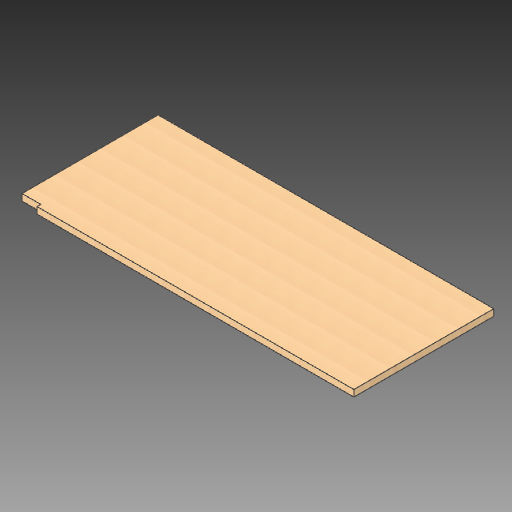
# Autodesk Inventor part: Причал фанера
Saved by Autodesk Inventor 2019 (Build 230136000, 136)
## iProperties
Created: 2018-10-10
Part Number: Причал фанера
Material: Ясень
Document SubType Name: Modeling
Designer: Андреев Н.Л.
Density: 0.641 g/cm^3
Appearance: Дверь — ясень
ШИРИНА: 371
ДЛИНА: 890
ТОЛЩВЫС: 17
Author: Андреев Н.Л.
Autodesk Inventor part; units mm, degrees
ref_plane "YZ Plane" through (0, 0, 0) normal (1, 0, 0) x (0, 1, 0)
ref_plane "XZ Plane" through (0, 0, 0) normal (0, 1, 0) x (-1, 0, 0)
ref_plane "XY Plane" through (0, 0, 0) normal (0, 0, 1) x (1, 0, 0)
sketch "Эскиз1" plane through (0, 0, 0) normal (0, 1, 0) x (-1, 0, 0)
  line L0 (0, 0) -> (890, 0)
  line L1 (890, 0) -> (890, 371)
  line L2 (890, 371) -> (0, 371)
  line L3 (0, 371) -> (0, 0)
  dimension "ШИРИНА" = 371
  dimension "ДЛИНА" = 890
  constraints: 8 end point, 2 parallel, 1 horizontal, 1 perpendicular
  measures "ШИРИНА" distance between parallel lines of L2 L0
  measures "ДЛИНА" distance between parallel lines of L3 L1
extrude "Выдавливание1" add sketch "Эскиз1" against normal blind 17.4
sketch "Эскиз2" plane through (-890, 0, 371) normal (0, 0, 1) x (1, 0, 0)
  line L0 (0, 0) -> (890, 0) construction
  line L1 (0, 0) -> (0, -17.4) construction
  line L2 (890, -17.4) -> (0, -17.4) construction
  line L3 (890, 0) -> (890, -17.4) construction
  line L4 (0, 0) -> (50, 0)
  line L5 (50, 0) -> (50, -17.4)
  line L6 (50, -17.4) -> (0, -17.4)
  line L7 (0, -17.4) -> (0, 0)
  point P0 (890, 0)
  dimension "d4" = 50
  constraints: 8 end point, 2 parallel, 1 horizontal, 1 perpendicular, 1 point on line
  measures "d4" distance of L5.end L6.end
extrude "Выдавливание2" cut sketch "Эскиз2" against normal blind 10
equation "\"ДЛИНА\" = пДлПроступи - пОтступПодступ"
equation "\"ТОЛЩВЫС\" = пТолПодступенка"
equation "\"d4\" = пОтступШипа"
equation "\"d5\" = пШипПодступ"
equation "\"пДлПроступи\" = 900"
equation "\"пПодъем\" = 162.5"
equation "\"пХод\" = 296.8"
equation "\"пЭффШаг\" = 621.8"
equation "\"пСвес\" = 30.2"
equation "\"пОтступСтен\" = 5"
equation "\"пДиаг\" = 338.3733"
equation "\"пШирПроступи\" = 327"
equation "\"пТолПодступенка\" = 17.4"
equation "\"пШипПодступ\" = 10"
equation "\"пОтступШипа\" = 50"
equation "\"пГлубПаза\" = 12"
equation "\"пОтступПодступ\" = 10"
equation "\"пОтступОтСтен\" = 5"
equation "\"пТолПричала\" = 17.4"
